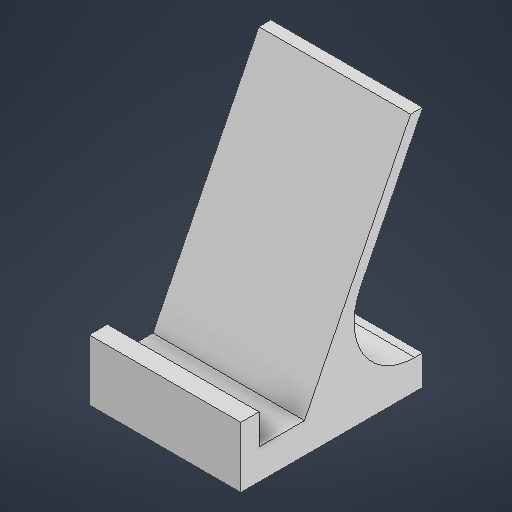
# Autodesk Inventor part: hahahaurwelcome
Saved by Autodesk Inventor 2026 (Build 300175050, 175E)
## iProperties
Created: 2025-11-03
Part Number: hahahaurwelcome
Material: Generic
Document SubType Name: Modeling
Designer: ua
Density: 1 g/cm^3
Appearance: Default
Author: ua
Autodesk Inventor part; units mm, degrees
ref_plane "YZ Plane" through (0, 0, 0) normal (1, 0, 0) x (0, 1, 0)
ref_plane "XZ Plane" through (0, 0, 0) normal (0, 1, 0) x (-1, 0, 0)
ref_plane "XY Plane" through (0, 0, 0) normal (0, 0, 1) x (1, 0, 0)
sketch "Sketch1" plane through (0, 0, 0) normal (0, 1, 0) x (-1, 0, 0)
  line L0 (38.1, 38.1) -> (-38.1, 38.1)
  line L1 (-38.1, 38.1) -> (-38.1, -38.1)
  line L2 (-38.1, -38.1) -> (38.1, -38.1)
  line L3 (38.1, -38.1) -> (38.1, 38.1)
  line L4 (38.1, 38.1) -> (-38.1, -38.1) construction
  line L5 (-38.1, 38.1) -> (38.1, -38.1) construction
  point P0 (0, 0)
  dimension "d0" = 76.2
  dimension "d1" = 76.2
  constraints: 12 end point, 2 midpoint, 2 parallel, 1 horizontal, 1 perpendicular
  measures "d0" distance of L2.end L1.end
  measures "d1" distance of L1.end L0.end
extrude "Extrusion1" add sketch "Sketch1" along normal blind 101.6
sketch "Sketch2" plane through (38.1, 0, 38.1) normal (1, 0, 0) x (0, 0, -1)
  line L0 (31.7497, 12.5069) -> (76.1457, 101.4069)
  line L1 (76.1457, 101.4069) -> (165.0457, 101.4069) construction
  line L2 (76.1457, 12.5069) -> (31.7497, 12.5069)
  line L3 (76.1457, 12.5069) -> (78.6857, 12.5069)
  line L4 (78.6857, 12.5069) -> (78.6857, 101.4069)
  line L5 (78.6857, 101.4069) -> (76.1457, 101.4069)
  point P0 (38.1, 0)
  dimension "d8" = 88.9
  dimension "d10" = 2.54
  dimension "d11" = 88.9
  constraints: 12 end point, 2 horizontal, 1 parallel, 1 perpendicular
  measures "d8" distance of L0.end L2.start
  measures "d10" distance of L5.end L4.end
  measures "d11" distance of L4.end L3.end
extrude "Extrusion2" cut sketch "Sketch2" against normal blind 101.6
fillet "Fillet1" radius 25.4 1 edges at (0, 12.5069, 6.3503)
sketch "Sketch3" plane through (38.1, 0, 38.1) normal (1, 0, 0) x (0, 0, -1)
  line L0 (7.62, 25.4) -> (0, 25.4)
  line L1 (26.67, 12.7) -> (7.62, 12.7)
  line L2 (26.67, 12.7) -> (71.066, 101.6)
  line L3 (76.2, 101.6) -> (0, 101.6) projected
  line L4 (0, 25.4) -> (-2.0413, 103.693)
  line L5 (-2.0413, 103.693) -> (71.066, 101.6)
  line L6 (7.62, 12.7) -> (7.62, 25.4)
  line L7 (50.1015, 49.2551) -> (76.1457, 101.4069) projected
  point P0 (38.1, 0)
  dimension "d15" = 7.62
  dimension "d17" = 19.05
  constraints: 12 end point, 1 parallel, 1 point on line, 1 vertical
  measures "d15" distance of L0.end L0.start
  measures "d17" distance of L1.end L1.start
extrude "Extrusion3" cut sketch "Sketch3" against normal blind 101.6
sketch "Sketch4" plane through (0, 0, 0) normal (0, -1, 0) x (1, 0, 0)
  line L0 (50.8, 45.6457) -> (25.4, 45.6457)
  line L1 (25.4, 45.6457) -> (25.4, -45.6457)
  line L2 (25.4, -45.6457) -> (50.8, -45.6457)
  line L3 (50.8, -45.6457) -> (50.8, 45.6457)
  line L4 (38.1, -32.966) -> (38.1, 11.43) projected
  line L5 (50.8, 45.6457) -> (25.4, -45.6457) construction
  line L6 (25.4, 45.6457) -> (50.8, -45.6457) construction
  point P0 (0, 0)
  point P1 (38.1, 0)
  dimension "d21" = 25.4
  constraints: 12 end point, 2 midpoint, 2 parallel, 1 horizontal, 1 perpendicular, 1 point on line
  measures "d21" distance of L2.end L1.end
extrude "Extrusion4" cut sketch "Sketch4" against normal blind 101.6
body "Solid1"
